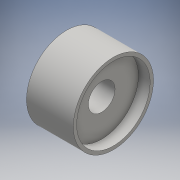
# Autodesk Inventor part: Bearing
Saved by Autodesk Inventor 2016 (Build 200138000, 138)
## iProperties
Created: 2016-01-06
Part Number: Bearing
Material: Generic
Document SubType Name: Modeling
Designer: m2memari
Density: 1 g/cm^3
Appearance: Default
Author: m2memari
Autodesk Inventor part; units mm, degrees
ref_plane "YZ Plane" through (0, 0, 0) normal (1, 0, 0) x (0, 1, 0)
ref_plane "XZ Plane" through (0, 0, 0) normal (0, 1, 0) x (-1, 0, 0)
ref_plane "XY Plane" through (0, 0, 0) normal (0, 0, 1) x (1, 0, 0)
sketch "Sketch1" plane through (0, 0, 0) normal (1, 0, 0) x (0, 1, 0)
  circle A0 centre (0, 0) radius 4
  circle A1 centre (0, 0) radius 11
  dimension "d0" = 8
  dimension "d1" = 22
  constraints: 2 centre point, 2 coincident
  measures "d0" diameter of A0
  measures "d1" diameter of A1
extrude "Extrusion1" add sketch "Sketch1" along normal mid plane 7
ref_plane "Work Plane1" through (0, 0, 0) normal (-1, 0, 0) x (0, 0, 1)
sketch "Sketch3" plane through (0, 0, 0) normal (-1, 0, 0) x (0, 0, 1)
  circle A0 centre (0, 0) radius 12
  circle A1 centre (0, 0) radius 11
  dimension "d5" = 24
  dimension "d6" = 22
  constraints: 2 centre point, 2 coincident
  measures "d5" diameter of A0
  measures "d6" diameter of A1
extrude "Extrusion2" add sketch "Sketch3" along normal mid plane 14
equation "\"d0\" = BearingShaftDiameter"
equation "\"d2\" = BearingWidth"
equation "\"d5\" = BearingDiameter"
equation "\"d7\" = BearingSiliconeWidth"
equation "\"d4\" = -0.5 * BearingWidth"
equation "\"BearingShaftDiameter\" = 8"
equation "\"BearingWidth\" = 7"
equation "\"BearingDiameter\" = 24"
equation "\"BearingSiliconeWidth\" = 14"
body "Solid1"
